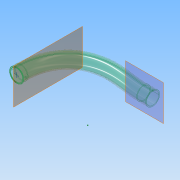
# Autodesk Inventor part: Top_LHS Pipe 2
Saved by Autodesk Inventor 2018.1 (Build 221171000, 171)
## iProperties
Created: 2019-03-19
Part Number: Top_LHS Pipe 2
Material: PMMA Plastic
Document SubType Name: Modeling
Designer: James
Density: 1.188 g/cm^3
Appearance: Clear - Green 1
Mass: 181.924 g
Surface Area: 1029.82 cm^2
Volume: 153.134 cm^3
Author: James
Autodesk Inventor part; units mm, degrees
ref_plane "XY Plane" through (0, 0, 0) normal (0, 0, 1) x (1, 0, 0)
sketch "Sketch2" plane through (0, 0, 0) normal (1, 0, 0) x (0, 1, 0)
  circle A0 centre (0, 0) radius 20
  circle A1 centre (0, 0) radius 23
  dimension "d2" = 40
  dimension "d3" = 46
  constraints: 2 centre point, 2 coincident
  measures "d2" diameter of A0
  measures "d3" diameter of A1
sketch3d "3D Sketch1"
  spline S0 degree 4 poles (0, 0, 0) (-80, 0, 0) (-80, 0, 26) (-233, 0, 26) (-233, -168, 26) knots 1 1 1 1 1 2 2 2 2 2
  dimension "d4" = 80
  dimension "d6" = 153
  dimension "d7" = 168
  dimension "d24" = 26
sweep "Sweep1" add profiles "Sketch2" path "3D Sketch1"
sketch "Sketch3" plane through (0, 0, 0) normal (1, 0, 0) x (0, 0, -1)
  spline S0 degree 6 poles (0, 20) (33.2309, 20) (38.0022, -21.091) (0, -54.9823) (-38.0022, -21.091) (-33.2309, 20) (0, 20) knots 0 0 0 0 0 0 0 1 1 1 1 1 1 1 weights 1.669078 1.03673 1.038347 0.853534 1.038347 1.03673 1.669078 projected
  circle A0 centre (0, 0) radius 23 projected
  point P0 (0, 23)
  constraints: 1 vertical alignment, 1 other
extrude "Extrusion1" add sketch "Sketch3" along normal blind 30
ref_plane "Work Plane1" through (0, 0, 0) normal (0, 1, 0) x (1, 0, 0)
sketch "Sketch4" plane through (0, 0, 0) normal (0, 1, 0) x (1, 0, 0)
  line L0 (30, -23) -> (30, 23) projected
  line L1 (0, 23) -> (0, -23) projected
  point P0 (0, 0)
  point P1 (7.5, 0)
  point P2 (30, 0)
  point P3 (0, 0)
  dimension "d23" = 7.5
  constraints: 1 horizontal alignment, 1 midpoint
  measures "d23" distance of point (7.5, 0) point (0, 0)
hole "Hole1" at (7.5, 0, 0) direction (0, 1, 0) diameter 4.5 end through all
sketch "Sketch5" plane through (-233, -168, 26) normal (0, -1, 0) x (1, 0, 0)
  spline S0 degree 6 poles (-19.8922, 2.074) (-23.3382, -30.9777) (17.0365, -39.9845) (54.6859, -5.7016) (24.918, 35.6103) (-16.4462, 35.1257) (-19.8922, 2.074) knots 0 0 0 0 0 0 0 1 1 1 1 1 1 1 weights 1.669078 1.03673 1.038347 0.853534 1.038347 1.03673 1.669078 projected
  circle A0 centre (0, 0) radius 23 projected
  point P0 (233, -26)
  point P1 (-22.8793, 2.3534)
  constraints: 2 other
extrude "Extrusion2" add sketch "Sketch5" along normal blind 15 contours S0 picked at (15.0567, 15.8447)
sketch "Sketch6" plane through (-233, -183, 26) normal (0, -1, 0) x (1, 0, 0)
  circle A0 centre (0, 0) radius 23 projected
  point P0 (233, -26)
  constraints: 1 coincident, 1 other
ref_plane "Work Plane2" through (-233, -183, 26) normal (1, 0, 0) x (0, 1, 0)
sketch "Sketch7" plane through (-233, -183, 26) normal (1, 0, 0) x (0, 1, 0)
  line L0 (0, 23) -> (0, -23) projected
  point P0 (183, -26)
  point P1 (8.5, 0)
  point P2 (0, 0)
  dimension "d27" = 8.5
  constraints: 1 horizontal alignment, 1 midpoint
  measures "d27" distance from line of point (8.5, 0) L0
hole "Hole2" at (-233, -174.5, 26) direction (1, 0, 0) diameter 4.5 end through all
body "Solid1"
